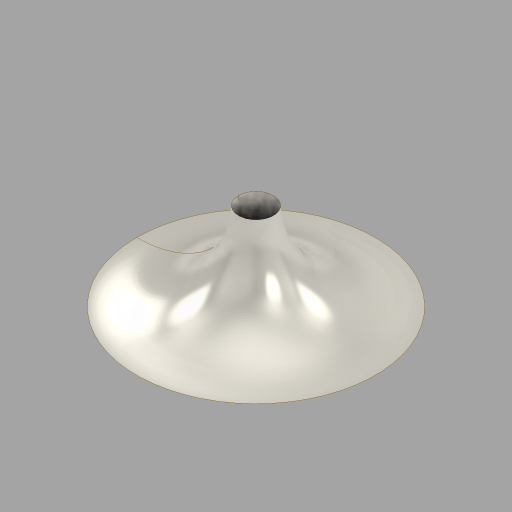
# Autodesk Inventor part: TorsionOscillator-Solder-1
Saved by Autodesk Inventor 2024 (Build 280153020, 153B)
## iProperties
Created: 2023-08-21
Part Number: TorsionOscillator-Solder-1
Material: Titanium
Document SubType Name: Modeling
Designer: schanen
Density: 4.51 g/cm^3
Appearance: Titanium
Author: schanen
Autodesk Inventor part; units mm, degrees
ref_plane "YZ Plane" through (0, 0, 0) normal (1, 0, 0) x (0, 1, 0)
ref_plane "XZ Plane" through (0, 0, 0) normal (0, 1, 0) x (-1, 0, 0)
ref_plane "XY Plane" through (0, 0, 0) normal (0, 0, 1) x (1, 0, 0)
sketch "Sketch1" plane through (0, 0, 0) normal (0, 0, 1) x (1, 0, 0)
  line L0 (-0.6, 0) -> (-0.6, 3)
  line L1 (-0.6, 0) -> (-4.1, 0)
  ellipse E0 centre (-4.1, 3) end of major axis (-4.1, 0) minor radius 3.5
  line L2 (0, -1.2) -> (0, 7.2) projected
  point P0 (0, 0)
  dimension "d0" = 4.1
  dimension "d1" = 0.6
  dimension "d2" = 3
  constraints: 4 end point, 1 horizontal, 1 vertical, 4 other
  measures "d0" distance of point (0, 0) L1.end
  measures "d1" distance from line of point (0, 0) L0
  measures "d2" distance of L0.start L0.end
revolve "Revolution1" add sketch "Sketch1" angle 360 about axis through (0, -10, 0) along (0, 1, 0) contours L1 E0 L0
body "Solid1"
